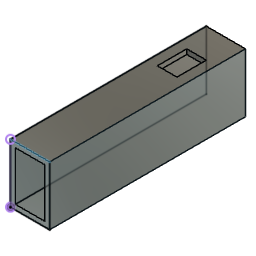
parte de abajo (Autodesk Fusion 360 design; units mm, degrees)
Autodesk Fusion 360 part; units mm, degrees
sketch "Boceto1" plane through (0, 0, 0) normal (0, 0, 1) x (1, 0, 0)
  line L0 (0, 0) -> (20, 0)
  line L1 (20, 0) -> (20, 100)
  line L2 (20, 100) -> (0, 100)
  line L3 (0, 100) -> (0, 0)
  dimension "d1" = 20
  dimension "d2" = 100
  constraint horizontal L0
  constraint vertical L1
  constraint horizontal L2
  constraint vertical L3
  constraint coincident L0.start L3.end
  measures "d1" distance of L0.start L0.end
  measures "d2" distance of L0.start L2.end
sketch "Boceto2" plane through (0, 0, 0) normal (1, 0, 0) x (0, 1, 0)
  line L0 (0, 0) -> (100, 0)
  line L1 (100, 0) -> (100, 30)
  line L2 (100, 30) -> (0, 30)
  line L3 (0, 30) -> (0, 0)
  dimension "d3" = 100
  dimension "d4" = 30
  constraint horizontal L0
  constraint vertical L1
  constraint horizontal L2
  constraint vertical L3
  constraint coincident L0.start L3.end
  measures "d3" distance of L0.start L0.end
  measures "d4" distance of L0.end L1.end
sketch "Boceto3" plane through (0, 0, 0) normal (1, 0, 0) x (0, 1, 0)
sketch "Boceto4" plane through (0, 0, 0) normal (0, 1, 0) x (1, 0, 0)
  line L0 (0, 0) -> (20, 0)
  line L1 (20, 0) -> (20, -30)
  line L2 (20, -30) -> (0, -30)
  line L3 (0, -30) -> (0, 0)
  line L4 (0, -30) -> (0, 0)
  dimension "d5" = 20
  dimension "d6" = 30
  constraint horizontal L0
  constraint vertical L1
  constraint horizontal L2
  constraint vertical L3
  constraint coincident L0.start L3.end
  measures "d5" distance of L0.start L0.end
  measures "d6" distance of L2.end L0.start
sketch "Boceto5" plane through (0, 0, 0) normal (0, 0, 1) x (1, 0, 0)
extrude "Extruir1" add sketch "Boceto1" along normal blind 30
sketch "Boceto6" plane through (0, 100, 0) normal (0, 1, 0) x (-1, 0, 0)
  line L0 (-20, 0) -> (0, 0)
  line L1 (0, 0) -> (0, 30)
  line L2 (0, 30) -> (-20, 30)
  line L3 (-20, 30) -> (-20, 0)
  line L4 (-2.5, 2.5) -> (-17.5, 2.5)
  line L5 (-17.5, 2.5) -> (-17.5, 27.5)
  line L6 (-17.5, 27.5) -> (-2.5, 27.5)
  line L7 (-2.5, 27.5) -> (-2.5, 2.5)
  dimension "d9" = 25
  dimension "d10" = 15
  constraint horizontal L4
  constraint vertical L5
  constraint horizontal L6
  constraint vertical L7
  measures "d9" distance of L4.end L5.end
  measures "d10" distance of L4.start L4.end
extrude "Extruir2" cut sketch "Boceto6" against normal blind 20 contours L4 L5 L6 L7
hole "Agujero1" at (10.0437, 100, 28.1947) direction (0, -1, 0) diameter 1 depth 8 tip angle 118
hole "Agujero2" at (9.9089, 100, 1.7915) direction (0, -1, 0) diameter 1 depth 8 tip angle 118
extrude "Extruir3" cut 1 faces at (7.5, 80, 10.8333) along direction (0, -1, 0) blind 79
extrude "Extruir4" cut 1 faces at (7.5, 1, 10.8333) along direction (0, -1, 0) blind 105
sketch "Boceto7" plane through (20, 0, 0) normal (1, 0, 0) x (0, 1, 0)
  line L0 (0, 0) -> (100, 0)
  line L1 (100, 0) -> (100, 30)
  line L2 (100, 30) -> (0, 30)
  line L3 (0, 30) -> (0, 0)
sketch "Boceto8" plane through (0, 0, 30) normal (0, 0, 1) x (-1, 0, 0)
  line L0 (0, -100) -> (0, 0)
  line L1 (0, 0) -> (-20, 0)
  line L2 (-20, 0) -> (-20, -100)
  line L3 (-20, -100) -> (0, -100)
  line L4 (-20, -100) -> (-20, 0)
  line L5 (-15, -70) -> (-5, -70)
  line L6 (-5, -70) -> (-5, -80)
  line L7 (-5, -80) -> (-15, -80)
  line L8 (-15, -80) -> (-15, -70)
  line L9 (-5, -80) -> (-15, -80)
  line L10 (-15, -80) -> (-15, -70)
  line L11 (-15, -70) -> (-5, -70)
  line L12 (-5, -70) -> (-5, -80)
  dimension "d23" = 100
  dimension "d24" = 20
  constraint horizontal L5
  constraint vertical L6
  constraint horizontal L7
  constraint vertical L8
  constraint horizontal L9
  constraint vertical L10
  constraint horizontal L11
  constraint vertical L12
  measures "d23" distance of L2.end L1.end
  measures "d24" distance of L0.start L2.end
extrude "Extruir5" cut sketch "Boceto8" against normal blind 7 contours L5 L6 L7 L8 L9 L10 L11 L12
sketch "Boceto9" plane through (0, 0, 30) normal (0, 0, 1) x (-1, 0, 0)
  line L0 (-15, -80) -> (-15, -70)
  line L1 (-15, -70) -> (-5, -70)
  line L2 (-5, -70) -> (-5, -80)
  line L3 (-5, -80) -> (-15, -80)
  line L4 (0, -100) -> (0, 0)
  line L5 (0, 0) -> (-20, 0)
  line L6 (-20, 0) -> (-20, -100)
  line L7 (-20, -100) -> (0, -100)
  line L8 (-15, -80) -> (-5, -80)
  line L9 (-5, -80) -> (-5, -85)
  line L10 (-5, -85) -> (-15, -85)
  line L11 (-15, -85) -> (-15, -80)
  constraint horizontal L8
  constraint vertical L9
  constraint horizontal L10
  constraint vertical L11
  constraint coincident L0.start L3.end
extrude "Extruir6" cut sketch "Boceto9" against normal blind 4 contours L3 L8 L9 L10 L11
